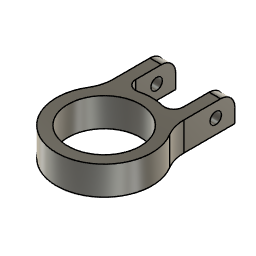
Drum Frame Stabiliser Bracket v0 (Autodesk Fusion 360 design; units mm, degrees)
Autodesk Fusion 360 part; units mm, degrees
sketch "Sketch1" plane through (0, 0, 0) normal (0, 0, 1) x (1, 0, 0)
  circle A0 centre (0, 0) radius 19
  line L0 (0, 0) -> (0, 68.0684) construction
  line L1 (-12.5, 21.6506) -> (-12.5, 50)
  line L2 (-18.5, 50) -> (-12.5, 50)
  line L3 (12.5, 50) -> (18.5, 50)
  line L4 (-18.5, 50) -> (-18.5, 16.8152)
  line L5 (12.5, 21.6506) -> (12.5, 50)
  line L6 (18.5, 50) -> (18.5, 16.8152)
  arc A1 (-18.5, 16.8152) -> (18.5, 16.8152) centre (0, 0) ccw
  arc A2 (12.5, 21.6506) -> (-12.5, 21.6506) centre (0, 0) ccw
  dimension "d1" = 38
  dimension "d3" = 12.5
  dimension "d5" = 6
  constraint coincident A0.centre L0.start
  constraint vertical L0
  constraint parallel L0 L1
  constraint parallel L1 L4
  constraint parallel L1 L6
  constraint perpendicular L2 L6
  constraint collinear L2 L3
  constraint concentric A0 A1
  constraint coincident L5.start A1
  constraint concentric A1 A2
  measures "d1" diameter of A0
  measures "d3" distance of L0 L1
  measures "d5" distance of L1 L4
extrude "Extrude1" add sketch "Sketch1" along normal blind 15
fillet "Fillet1" radius 20 1 edges at (-18.5, 16.8152, 7.5)
fillet "Fillet2" radius 20 1 edges at (18.5, 16.8152, 7.5)
fillet "Fillet3" radius 5 1 edges at (-12.5, 21.6506, 7.5)
fillet "Fillet4" radius 5 1 edges at (12.5, 21.6506, 7.5)
sketch "Sketch2" plane through (18.5, 0, 0) normal (1, 0, 0) x (0, 1, 0)
  line L0 (23.297, 15) -> (23.297, 0)
  line L1 (23.297, 0) -> (50, 0)
  line L2 (50, 0) -> (50, 15)
  line L3 (50, 15) -> (23.297, 15)
  point P0 (40, 7.5)
  dimension "d17" = 7.5
  dimension "d18" = 10
  measures "d17" distance of L3 P0
  measures "d18" distance of L2 P0
hole "Hole1" at (18.5, 40, 7.5) direction (-1, 0, 0) diameter 6 depth 70 tip angle 118
fillet "Fillet5" radius 7.5 2 edges at (15.5, 50, 15) (-15.5, 50, 15)
